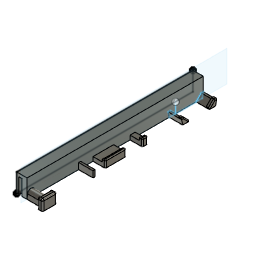
3dtoolholder v4 (Autodesk Fusion 360 design; units mm, degrees)
Autodesk Fusion 360 part; units mm, degrees
sketch "Schizzo2" plane through (0, 0, 0) normal (0, 1, 0) x (1, 0, 0)
  line L0 (0, 0) -> (2, 0)
  line L1 (2, 0) -> (2, -30)
  line L2 (2, -30) -> (0, -30)
  line L3 (0, -30) -> (0, 0)
  line L4 (2, -30) -> (5, -30)
  line L5 (5, -30) -> (5, -15)
  line L6 (5, -15) -> (2, -15)
  line L7 (2, -15) -> (2, -30)
  line L8 (5, -30) -> (10, -30)
  line L9 (10, -30) -> (10, 0)
  line L10 (10, 0) -> (5, 0)
  line L11 (5, 0) -> (5, -30)
  dimension "d1" = 2
  dimension "d2" = 30
  dimension "d3" = 3
  dimension "d4" = 30
  dimension "d5" = 5
  dimension "d44" = 15
  constraint horizontal L0
  constraint vertical L1
  constraint horizontal L2
  constraint vertical L3
  constraint coincident L0.start L3.end
  constraint horizontal L4
  constraint vertical L5
  constraint horizontal L6
  constraint vertical L7
  constraint horizontal L8
  constraint vertical L9
  constraint horizontal L10
  constraint vertical L11
  measures "d1" distance of L0.start L0.end
  measures "d2" distance of L0.start L2.end
  measures "d3" distance of L5.end L6.end
  measures "d4" distance of L8.end L9.end
  measures "d5" distance of L4.end L8.end
  measures "d44" distance of L4 L6
extrude "Estrusione1" add sketch "Schizzo2" along normal blind 200
sketch "Schizzo3" plane through (10, 0, 0) normal (1, 0, 0) x (0, 1, 0)
  line L0 (0, 30) -> (0, 0)
  line L1 (0, 0) -> (200, 0)
  line L2 (200, 0) -> (200, 30)
  line L3 (200, 30) -> (0, 30)
  line L4 (0, 30) -> (10, 30)
  circle A0 centre (10, 4) radius 3.5
  line L5 (6, 0) -> (6.5245, 4.413)
  line L6 (14, 0) -> (13.4755, 4.413)
  line L7 (6, 0) -> (14, 0)
  dimension "d8" = 7
  constraint coincident L0.start L3.end
  constraint coincident L3 L4.end
  constraint perpendicular L0 L4
  constraint coincident A0 L5.end
  constraint tangent A0 L5
  constraint coincident A0 L6.end
  constraint tangent A0 L6
  constraint horizontal L7
  measures "d8" diameter of A0
extrude "Estrusione2" add sketch "Schizzo3" along normal blind 13 contours L1 A0 L5 L6 L7 | A0
sketch "Schizzo4" plane through (23, 0, 0) normal (1, 0, 0) x (0, 1, 0)
  line L0 (3, 0) -> (17, 0)
  line L1 (17, 0) -> (17, 10)
  line L2 (17, 10) -> (3, 10)
  line L3 (3, 10) -> (3, 0)
  constraint horizontal L0
  constraint vertical L1
  constraint horizontal L2
  constraint vertical L3
extrude "Estrusione4" add sketch "Schizzo4" along normal blind 5
fillet "Raccordo3" radius 1.5 8 edges at (23, 10, 10) (25.5, 17, 10) (28, 10, 10) (25.5, 3, 10) (28, 3, 5) (23, 3, 5) (28, 17, 5) (23, 17, 5)
sketch "Schizzo5" plane through (10, 0, 0) normal (1, 0, 0) x (0, 1, 0)
  line L0 (13.4755, 4.413) -> (14, 0)
  line L1 (14, 0) -> (200, 0)
  line L2 (200, 0) -> (200, 30)
  line L3 (200, 30) -> (0, 30)
  line L4 (0, 30) -> (0, 0)
  line L5 (0, 0) -> (6, 0)
  line L6 (6, 0) -> (6.5245, 4.413)
  arc A0 (13.4755, 4.413) -> (6.5245, 4.413) centre (10, 4) ccw
sketch "Schizzo6" plane through (10, 0, 0) normal (1, 0, 0) x (0, 1, 0)
  line L0 (70, 0) -> (70, 4)
  line L1 (70, 0) -> (90, 0)
  line L2 (90, 0) -> (106, 0)
  line L3 (106, 0) -> (111, 0)
  line L4 (111, 0) -> (111, 4)
  line L5 (90, 0) -> (90, 4)
  line L6 (106, 0) -> (106, 4)
  line L7 (111, 4) -> (106, 4)
  line L8 (90, 4) -> (70, 4)
  dimension "d22" = 20
  dimension "d23" = 16
  dimension "d24" = 5
  constraint vertical L0
  constraint perpendicular L0 L1
  constraint parallel L1 L2
  constraint parallel L2 L3
  constraint perpendicular L3 L4
  constraint perpendicular L0 L7
  constraint coincident L5.end L7
  constraint perpendicular L5 L7
  constraint perpendicular L6 L7
  constraint collinear L7 L8
  measures "d22" distance of L0.start L1.end
  measures "d23" distance of L1.end L2.end
  measures "d24" distance of L2.end L3.end
extrude "Estrusione5" add sketch "Schizzo6" along normal blind 9
sketch "Schizzo7" plane through (19, 0, 0) normal (1, 0, 0) x (0, 1, 0)
  line L0 (70, 0) -> (90, 0)
  line L1 (90, 0) -> (90, 4)
  line L2 (90, 4) -> (70, 4)
  line L3 (70, 4) -> (70, 0)
  line L4 (70, 0) -> (90, 0)
  line L5 (90, 0) -> (90, 7)
  line L6 (90, 7) -> (70, 7)
  line L7 (70, 7) -> (70, 0)
  line L8 (106, 0) -> (111, 0)
  line L9 (111, 0) -> (111, 7)
  line L10 (111, 7) -> (106, 7)
  line L11 (106, 7) -> (106, 0)
  constraint horizontal L4
  constraint vertical L5
  constraint horizontal L6
  constraint vertical L7
  constraint coincident L0.start L3.end
  constraint horizontal L8
  constraint vertical L9
  constraint horizontal L10
  constraint vertical L11
extrude "Estrusione6" add sketch "Schizzo7" along normal blind 3
fillet "Raccordo4" radius 1 12 edges at (19, 108.5, 7) (22, 108.5, 7) (22, 80, 7) (19, 80, 7) (20.5, 90, 7) (20.5, 106, 7) (20.5, 111, 7) (22, 106, 3.5) (22, 111, 3.5) (22, 90, 3.5) (20.5, 70, 7) (22, 70, 3.5)
sketch "Schizzo8" plane through (10, 0, 0) normal (1, 0, 0) x (0, 1, 0)
  line L0 (150, 0) -> (150, 10)
  line L1 (150, 0) -> (170, 0)
  line L2 (170, 0) -> (175, 5)
  line L3 (145, 5) -> (150, 0)
  line L4 (145, 5) -> (143, 5)
  line L5 (148, 0) -> (150, 0)
  line L6 (175, 5) -> (177, 5)
  line L7 (170, 0) -> (172, 0)
  line L8 (143, 5) -> (144, 0)
  line L9 (144, 0) -> (148, 0)
  line L10 (177, 5) -> (176, 0)
  line L11 (176, 0) -> (172, 0)
  dimension "d31" = 20
  constraint vertical L0
  constraint perpendicular L0 L1
  constraint horizontal L4
  constraint perpendicular L0 L5
  constraint horizontal L6
  constraint parallel L1 L7
  constraint parallel L5 L9
  constraint parallel L7 L11
  measures "d31" distance of L0.start L1.end
extrude "Estrusione8" add sketch "Schizzo8" along normal blind 10
sketch "Schizzo9" plane through (20, 0, 0) normal (1, 0, 0) x (0, 1, 0)
  line L0 (170, 0) -> (176, 0)
  line L1 (176, 0) -> (177, 5)
  line L2 (177, 5) -> (175, 5)
  line L3 (175, 5) -> (170, 0)
  line L4 (143, 5) -> (143, 6)
  line L5 (143, 6) -> (145, 6)
  line L6 (145, 6) -> (150, 1)
  line L7 (150, 1) -> (150, 0)
  line L8 (143, 5) -> (144, 0)
  line L9 (144, 0) -> (150, 0)
  line L10 (170, 0) -> (170, 1)
  line L11 (170, 1) -> (175, 6)
  line L12 (175, 6) -> (177, 6)
  line L13 (177, 6) -> (177, 5)
  line L14 (176, 0) -> (177, 5)
  line L15 (170, 0) -> (176, 0)
  constraint vertical L4
  constraint perpendicular L4 L5
  constraint perpendicular L5 L7
  constraint perpendicular L7 L9
  constraint coincident L0.start L3.end
  constraint perpendicular L0 L10
  constraint parallel L3 L11
  constraint parallel L2 L12
  constraint coincident L1.end L2.start
  constraint perpendicular L2 L13
  constraint coincident L0.end L1.start
extrude "Estrusione9" add sketch "Schizzo9" along normal blind 3
fillet "Raccordo5" radius 1 4 edges at (23, 144, 6) (23, 147.5, 3.5) (23, 176, 6) (23, 172.5, 3.5)
sketch "Schizzo10" plane through (0, 200, 0) normal (0, 1, 0) x (-1, 0, 0)
  line L0 (0, 30) -> (-10, 30)
  line L1 (-10, 30) -> (-10, 0)
  line L2 (-10, 0) -> (-5, 0)
  line L3 (-5, 0) -> (-5, 15)
  line L4 (-5, 15) -> (-2, 15)
  line L5 (-2, 15) -> (-2, 0)
  line L6 (-2, 0) -> (0, 0)
  line L7 (0, 0) -> (0, 30)
  line L8 (-12, 31) -> (4, 31)
  line L9 (4, 31) -> (4, -5)
  line L10 (4, -5) -> (-12, -5)
  line L11 (-12, -5) -> (-12, 31)
  constraint horizontal L8
  constraint vertical L9
  constraint horizontal L10
  constraint vertical L11
extrude "Estrusione10" cut sketch "Schizzo10" against normal blind 23 contours L0 L1 L2 L3 L4 L5 L6 L7 | L8 L9 L10 L11
sketch "Schizzo11" plane through (0, 0, 0) normal (0, -1, 0) x (1, 0, 0)
  line L0 (10, 30) -> (0, 30)
  line L1 (0, 30) -> (0, 0)
  line L2 (0, 0) -> (2, 0)
  line L3 (2, 0) -> (2, 15)
  line L4 (2, 15) -> (5, 15)
  line L5 (5, 15) -> (5, 0)
  line L6 (5, 0) -> (10, 0)
  line L7 (10, 0) -> (10, 30)
  line L8 (-2, 31) -> (12, 31)
  line L9 (12, 31) -> (12, -1)
  line L10 (12, -1) -> (-2, -1)
  line L11 (-2, -1) -> (-2, 31)
  constraint horizontal L8
  constraint vertical L9
  constraint horizontal L10
  constraint vertical L11
extrude "Estrusione11" cut sketch "Schizzo11" against normal blind 6 contours L0 L1 L2 L3 L4 L5 L6 L7
sketch "Schizzo12" plane through (0, 6, 0) normal (0, -1, 0) x (1, 0, 0)
  line L0 (10, 0) -> (10, 30)
  line L1 (10, 30) -> (0, 30)
  line L2 (0, 30) -> (0, 0)
  line L3 (0, 0) -> (2, 0)
  line L4 (2, 0) -> (2, 15)
  line L5 (2, 15) -> (5, 15)
  line L6 (5, 15) -> (5, 0)
  line L7 (5, 0) -> (10, 0)
  line L8 (-2, 31) -> (11, 31)
  line L9 (11, 31) -> (11, 18)
  line L10 (11, 18) -> (-2, 18)
  line L11 (-2, 18) -> (-2, 31)
  dimension "d45" = 13
  constraint horizontal L8
  constraint vertical L9
  constraint horizontal L10
  constraint vertical L11
  measures "d45" distance of L8.start L10.end
extrude "Estrusione12" cut sketch "Schizzo12" against normal blind 175 contours L0 L1 L2 L10
sketch "Schizzo13" plane through (0, 0, 0) normal (-1, 0, 0) x (0, -1, 0)
  line L0 (-6, 18) -> (-177, 18)
  line L1 (-177, 18) -> (-177, 0)
  line L2 (-177, 0) -> (-6, 0)
  line L3 (-6, 0) -> (-6, 18)
  line L4 (-177, 18) -> (-6, 18)
  line L5 (-6, 18) -> (-6, 0)
  line L6 (-6, 0) -> (-177, 0)
  line L7 (-177, 0) -> (-177, 18)
  constraint horizontal L4
  constraint vertical L5
  constraint horizontal L6
  constraint vertical L7
  constraint coincident L2.end L3.start
  constraint coincident L0.end L1.start
sketch "Schizzo14" plane through (10, 0, 0) normal (1, 0, 0) x (0, 1, 0)
  line L0 (56, 0) -> (58, 0)
  line L1 (58, 0) -> (58, 6)
  line L2 (58, 6) -> (56, 6)
  line L3 (56, 6) -> (56, 0)
  line L4 (70, 6) -> (70, 0)
  dimension "d48" = 12
  dimension "d49" = 2
  dimension "d50" = 6
  constraint horizontal L0
  constraint vertical L1
  constraint horizontal L2
  constraint vertical L3
  measures "d48" distance of L1 L4
  measures "d49" distance of L0.start L0.end
  measures "d50" distance of L0.start L2.end
extrude "Estrusione13" add sketch "Schizzo14" along normal blind 14
